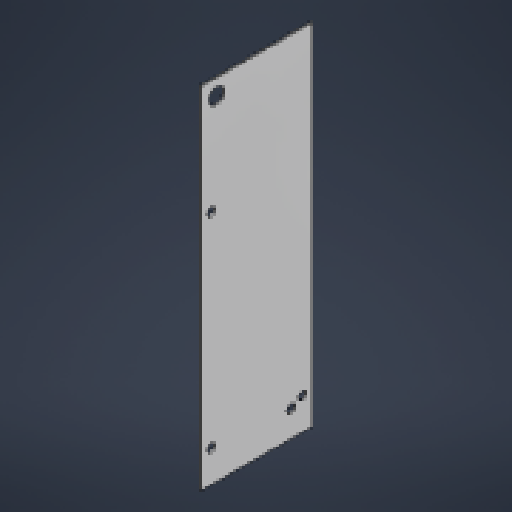
# Autodesk Inventor part: PLATE,BACK
Saved by Autodesk Inventor 2026.1 (Build 301233020, 233B)
## iProperties
Created: 2026-03-30
Part Number: PLATE,BACK
Material: Aluminum 6061
Document SubType Name: Sheet Metal
Designer: Owen L
Density: 2.7 g/cm^3
Sheet Metal Rule: Default
Appearance: Aluminum - Flat
Mass: 1097.51 g
Surface Area: 2621.74 cm^2
Volume: 406.485 cm^3
Author: Owen L
Autodesk Inventor part; units mm, degrees
ref_plane "YZ Plane" through (0, 0, 0) normal (1, 0, 0) x (0, 1, 0)
ref_plane "XZ Plane" through (0, 0, 0) normal (0, 1, 0) x (-1, 0, 0)
ref_plane "XY Plane" through (0, 0, 0) normal (0, 0, 1) x (1, 0, 0)
sketch "Sketch1" plane through (0, 0, 0) normal (1, 0, 0) x (0, 1, 0)
  line L0 (-317.5, 101.6) -> (317.5, 101.6)
  line L1 (317.5, 101.6) -> (317.5, -101.6)
  line L2 (317.5, -101.6) -> (-317.5, -101.6)
  line L3 (-317.5, -101.6) -> (-317.5, 101.6)
  line L4 (-317.5, 101.6) -> (317.5, -101.6) construction
  line L5 (317.5, 101.6) -> (-317.5, -101.6) construction
  point P0 (0, 0)
  dimension "d0" = 635
  dimension "d1" = 203.2
  measures "d0" distance of L1.end L2.end
  measures "d1" distance of L0.end L1.end
extrude "Plate1" add sketch "Sketch1" along normal blind 3.175
sketch "Sketch2" plane through (3.175, 0, 0) normal (1, 0, 0) x (0, 0, -1)
  circle A0 centre (-85.725, -254.7968) radius 11.1125
  circle A1 centre (84.455, -254.7968) radius 11.1125
  circle A2 centre (-85.725, 108.712) radius 11.1125
  circle A3 centre (84.455, 108.712) radius 11.1125
  circle A4 centre (-85.725, -254.7968) radius 11.938 construction
  circle A5 centre (84.455, -254.7968) radius 11.938 construction
  circle A6 centre (84.455, 108.712) radius 11.938 construction
  circle A7 centre (-85.725, 108.712) radius 11.938 construction
  line L0 (-101.6, -317.5) -> (-101.6, 317.5) projected
  circle A8 centre (64.0284, -269.8936) radius 12.7 construction
  circle A9 centre (64.0284, -269.8936) radius 11.1125
  point P0 (0, 0)
  point P1 (-138.1252, 190.5)
  dimension "d3" = 22.225
  dimension "d6" = 23.876
  dimension "d7" = 170.18
  dimension "d8" = 15.875
  dimension "d9" = 363.5088
  dimension "d10" = 81.788
  dimension "d11" = 25.4
  dimension "d12" = 25.4
  dimension "d13" = 150.5124
  constraints: 10 centre point, 7 equal radius, 5 coincident, 2 horizontal alignment, 2 vertical alignment
  measures "d3" diameter of A0
  measures "d6" diameter of A4
  measures "d7" distance of A0.centre A1.centre
  measures "d8" distance from line of L0 A0.centre
  measures "d9" distance of A2.centre A0.centre
  measures "d10" vertical distance of A2.centre point (-138.125, 190.5)
  measures "d11" diameter of A8
  measures "d12" distance of A1.centre A8.centre
  measures "d13" distance of A0.centre A8.centre
extrude "Cut1" cut sketch "Sketch2" against normal blind 3.175
sketch "Sketch3" plane through (3.175, 0, 0) normal (1, 0, 0) x (0, 0, -1)
  line L0 (-101.6, 269.875) -> (-101.6, 111.125) projected
  circle A0 centre (-73.025, 288.417) radius 11.1125
  point P0 (0, 0)
  point P1 (-101.6, 190.5)
  dimension "d16" = 22.225
  dimension "d17" = 97.917
  dimension "d18" = 28.575
  constraints: 1 centre point, 1 midpoint
  measures "d16" diameter of A0
  measures "d17" vertical distance of point (-101.6, 190.5) A0.centre
  measures "d18" distance from line of L0 A0.centre
extrude "Cut2" cut sketch "Sketch3" against normal blind 3.175
sketch "Sketch4" plane through (3.175, 0, 0) normal (1, 0, 0) x (0, 0, -1)
  circle A0 centre (64.0284, -269.8936) radius 11.1125 construction
  line L0 (64.0284, -269.8936) -> (57.8835, -245.2481) construction
  line L1 (64.0284, -269.8936) -> (52.1038, -292.3204) construction
  line L2 (64.0284, -269.8936) -> (86.0254, -282.5936) construction
  line L3 (64.0284, -269.8936) -> (64.0284, -241.3632) construction
  point P0 (0, 0)
  dimension "d21" = 25.4
  dimension "d22" = 14
  dimension "d23" = 28
  dimension "d24" = 60
  constraints: 8 end point, 2 equal length, 1 vertical
  measures "d21" distance of L0.start L0.end
  measures "d22" angle of L3 L0
  measures "d23" angle of L1 L3
  measures "d24" angle of L3 L2
hole "Hole1" at (3.175, -245.2481, -57.8835) at (3.175, -292.3204, -52.1038) at (3.175, -282.5936, -86.0254) direction (-1, 0, 0) diameter 5.6134 depth 3.175 tip angle 118 clearance for "Flat Head Machine Screw (82)" size "#10" standard "Ansi Unified Screw Threads"
equation "\"d14\" = Thickness"
equation "\"d19\" = Thickness"
equation "\"d30\" = Thickness"
equation "\"d2\" = Thickness"
equation "\"BendRadius\" = Thickness"
equation "\"BendReliefWidth\" = Thickness"
equation "\"BendReliefDepth\" = 0.5 * Thickness"
equation "\"CornerReliefSize\" = 4 * Thickness"
equation "\"MinimumRemnant\" = 2 * Thickness"
equation "\"TransitionRadius\" = BendRadius"
equation "\"JacobiRadiusSize\" = BendRadius"
equation "\"GapSize\" = Thickness"
equation "\"Thickness\" = 3.175"
body "Solid1"
